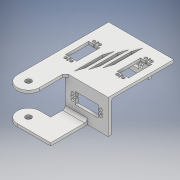
# Autodesk Inventor part: Rbiceps
Saved by Autodesk Inventor 2018 (Build 220112000, 112)
## iProperties
Created: 2018-02-07
Part Number: Rbiceps
Material: Plastique ABS
Document SubType Name: Modeling
Designer: Thomas
Density: 1.06 g/cm^3
Appearance: Lisse - Blanc
Mass: 118.74 g
Surface Area: 553.913 cm^2
Volume: 112.019 cm^3
Author: Thomas
Autodesk Inventor part; units mm, degrees
ref_plane "YZ Plane" through (0, 0, 0) normal (1, 0, 0) x (0, 1, 0)
ref_plane "XZ Plane" through (0, 0, 0) normal (0, 1, 0) x (-1, 0, 0)
ref_plane "XY Plane" through (0, 0, 0) normal (0, 0, 1) x (1, 0, 0)
sketch "Esquisse1" plane through (0, 0, 0) normal (0, 0, 1) x (1, 0, 0)
  line L0 (10, 0) -> (104.4, 0)
  line L1 (114.4, -10) -> (114.4, -105.15)
  line L2 (104.4, -115.15) -> (49, -115.15)
  line L3 (0, -115.15) -> (0, -10)
  line L4 (0, -115.15) -> (0, -160.65)
  line L5 (39, -160.65) -> (39, -125.15)
  arc A0 (0, -160.65) -> (39, -160.65) centre (19.5, -160.65) ccw
  line L6 (0, -10) -> (0, 0)
  line L7 (10, 0) -> (0, 0)
  line L8 (114.4, -10) -> (114.4, 0)
  line L9 (114.4, 0) -> (104.4, 0)
  line L10 (114.4, -105.15) -> (114.4, -115.15)
  line L11 (104.4, -115.15) -> (114.4, -115.15)
  line L12 (39, -125.15) -> (39, -115.15)
  line L13 (49, -115.15) -> (39, -115.15)
  dimension "d0" = 39
  dimension "d1" = 114.4
  dimension "d2" = 45.5
  dimension "d3" = 115.15
  constraints: 28 end point, 9 point on line, 5 vertical, 4 perpendicular, 2 horizontal, 2 parallel, 2 point on circle, 1 centre point
  measures "d0" distance of L4.end L5.start
  measures "d1" distance of L6.end L8.end
  measures "d2" distance of L5.start L12.end
  measures "d3" distance of L8.end L10.end
extrude "Extrusion1" add sketch "Esquisse1" along normal blind 5
sketch "Esquisse2" plane through (0, 0, 5) normal (0, 0, 1) x (1, 0, 0)
  line L0 (31.7, -46.85) -> (31.7, -87.85)
  line L1 (11.7, -87.85) -> (11.7, -46.85)
  line L2 (102.7, -26.7) -> (102.7, -67.7)
  line L3 (82.7, -67.7) -> (82.7, -26.7)
  line L4 (0, 0) -> (0, -160.65) projected
  line L5 (114.4, -115.15) -> (114.4, 0) projected
  circle A0 centre (16.7, -42.46) radius 2.5
  circle A1 centre (26.7, -42.46) radius 2.5
  circle A2 centre (16.7, -92.24) radius 2.5
  circle A3 centre (26.7, -92.24) radius 2.5
  circle A4 centre (87.7, -72.09) radius 2.5
  circle A5 centre (97.7, -72.09) radius 2.5
  circle A6 centre (87.7, -22.31) radius 2.5
  circle A7 centre (97.7, -22.31) radius 2.5
  circle A8 centre (19.5, -160.65) radius 5
  line L6 (114.4, 0) -> (0, 0) projected
  line L7 (39, -115.15) -> (114.4, -115.15) projected
  line L8 (22.7, -46.85) -> (22.7, -39.35)
  line L9 (22.7, -39.35) -> (20.7, -39.35)
  line L10 (20.7, -39.35) -> (20.7, -46.85)
  line L11 (93.7, -67.7) -> (93.7, -75.2)
  line L12 (91.7, -75.2) -> (91.7, -67.7)
  line L13 (93.7, -26.7) -> (93.7, -19.2)
  line L14 (93.7, -19.2) -> (91.7, -19.2)
  line L15 (91.7, -19.2) -> (91.7, -26.7)
  line L16 (11.7, -46.85) -> (20.7, -46.85)
  line L17 (31.7, -46.85) -> (22.7, -46.85)
  line L18 (22.7, -87.85) -> (22.7, -95.35)
  line L19 (22.7, -95.35) -> (20.7, -95.35)
  line L20 (20.7, -95.35) -> (20.7, -87.85)
  line L21 (11.7, -87.85) -> (20.7, -87.85)
  line L22 (22.7, -87.85) -> (31.7, -87.85)
  line L23 (82.7, -26.7) -> (91.7, -26.7)
  line L24 (93.7, -26.7) -> (102.7, -26.7)
  line L25 (82.7, -67.7) -> (91.7, -67.7)
  line L26 (93.7, -67.7) -> (102.7, -67.7)
  line L27 (91.7, -75.2) -> (93.7, -75.2)
  point P0 (0, -10)
  point P1 (114.4, -105.15)
  point P2 (114.4, -10)
  point P3 (39, -160.65)
  point P4 (104.4, 0)
  point P5 (10, 0)
  point P6 (49, -115.15)
  point P7 (104.4, -115.15)
  dimension "d7" = 11.7
  dimension "d8" = 11.7
  dimension "d9" = 20
  dimension "d10" = 20
  dimension "d11" = 41
  dimension "d12" = 41
  dimension "d13" = 10
  dimension "d14" = 19.5
  dimension "d16" = 5
  dimension "d18" = 5
  dimension "d20" = 10
  dimension "d21" = 5
  dimension "d22" = 5
  dimension "d26" = 10
  dimension "d28" = 5
  dimension "d31" = 5
  dimension "d32" = 10
  dimension "d33" = 5
  dimension "d36" = 5
  dimension "d37" = 10
  dimension "d41" = 9
  dimension "d43" = 4.39
  dimension "d44" = 4.39
  dimension "d45" = 5
  dimension "d46" = 7.5
  dimension "d47" = 7.5
  dimension "d48" = 9
  dimension "d49" = 9
  dimension "d50" = 9
  dimension "d51" = 5
  dimension "d52" = 4.39
  dimension "d53" = 4.39
  dimension "d54" = 7.5
  dimension "d55" = 9
  dimension "d56" = 9
  dimension "d57" = 4.39
  dimension "d58" = 4.39
  dimension "d59" = 5
  dimension "d60" = 9
  dimension "d61" = 9
  dimension "d62" = 7.5
  dimension "d63" = 4.39
  dimension "d64" = 4.39
  dimension "d65" = 5
  dimension "d168" = 41
  dimension "d169" = 41
  constraints: 48 end point, 9 centre point, 8 parallel, 4 horizontal, 3 collinear, 1 point on line
  measures "d7" distance between parallel lines of L1 L4
  measures "d8" distance between parallel lines of L5 L2
  measures "d9" distance of L0.end L1.start
  measures "d10" distance of L2.end L3.start
  measures "d11" distance of L0.start L0.end
  measures "d12" distance of L3.start L3.end
  measures "d13" diameter of A8
  measures "d14" distance of A8.centre point (39, -160.65)
  measures "d16" diameter of A2
  measures "d18" diameter of A3
  measures "d20" distance of A3.centre A2.centre
  measures "d21" diameter of A0
  measures "d22" diameter of A1
  measures "d26" distance of A1.centre A0.centre
  measures "d28" diameter of A5
  measures "d31" diameter of A4
  measures "d32" distance of A5.centre A4.centre
  measures "d33" diameter of A7
  measures "d36" diameter of A6
  measures "d37" distance of A7.centre A6.centre
  measures "d41" distance of L1.end L10.end
  measures "d43" distance from line of L16 A0.centre
  measures "d44" distance from line of L17 A1.centre
  measures "d45" horizontal distance of L1.end A0.centre
  measures "d46" distance of L8.start L8.end
  measures "d47" distance of L18.start L18.end
  measures "d48" distance of L1.start L20.end
  measures "d49" distance of L18.start L0.end
  measures "d50" distance of L0.start L8.start
  measures "d51" horizontal distance of A2.centre L1.start
  measures "d52" distance from line of L21 A2.centre
  measures "d53" distance from line of L22 A3.centre
  measures "d54" distance of L11.start L11.end
  measures "d55" distance of L3.start L12.end
  measures "d56" distance of L11.start L2.end
  measures "d57" distance from line of L25 A4.centre
  measures "d58" distance from line of L26 A5.centre
  measures "d59" distance from line of A4.centre L3
  measures "d60" distance of L3.end L15.end
  measures "d61" distance of L13.start L2.start
  measures "d62" distance of L14.end L15.end
  measures "d63" distance from line of L23 A6.centre
  measures "d64" distance from line of L24 A7.centre
  measures "d65" distance from line of L2 A7.centre
  measures "d168" distance of L1.start L1.end
  measures "d169" distance of L2.start L2.end
extrude "Extrusion2" cut sketch "Esquisse2" against normal blind 5
sketch "Esquisse3" plane through (39, -115.15, 0) normal (0, -1, 0) x (1, 0, 0)
  line L0 (0, 0) -> (75.4, 0) projected
  line L1 (0, 0) -> (75.4, 0)
  line L2 (75.4, 0) -> (75.4, -54.86)
  line L3 (75.4, -54.86) -> (0, -54.86)
  line L4 (0, -54.86) -> (0, 0)
  point P0 (-39, 0)
  dimension "d68" = 54.86
  constraints: 8 end point, 2 parallel, 1 horizontal, 1 perpendicular
  measures "d68" distance of L1.end L2.end
extrude "Extrusion3" add sketch "Esquisse3" against normal blind 5
sketch "Esquisse4" plane through (0, 0, 5) normal (0, 0, 1) x (1, 0, 0)
  line L0 (44.7, -55.15) -> (49.7, -40.15)
  line L1 (49.7, -40.15) -> (49.7, -90.15)
  line L2 (49.7, -90.15) -> (44.7, -105.15)
  line L3 (44.7, -105.15) -> (44.7, -55.15)
  line L4 (0, 0) -> (0, -160.65) projected
  line L5 (54.7, -40) -> (59.7, -25)
  line L6 (59.7, -25) -> (59.7, -75)
  line L7 (59.7, -75) -> (54.7, -90)
  line L8 (54.7, -90) -> (54.7, -40)
  line L9 (64.7, -25) -> (69.7, -10)
  line L10 (69.7, -10) -> (69.7, -60)
  line L11 (69.7, -60) -> (64.7, -75)
  line L12 (64.7, -75) -> (64.7, -25)
  line L13 (114.4, 0) -> (0, 0) projected
  line L14 (39, -115.15) -> (114.4, -115.15) projected
  dimension "d71" = 50
  dimension "d72" = 50
  dimension "d73" = 15
  dimension "d74" = 15
  dimension "d75" = 5
  dimension "d78" = 44.7
  dimension "d79" = 50
  dimension "d80" = 50
  dimension "d81" = 15
  dimension "d82" = 15
  dimension "d83" = 5
  dimension "d84" = 54.7
  dimension "d85" = 50
  dimension "d86" = 50
  dimension "d87" = 15
  dimension "d88" = 15
  dimension "d89" = 5
  dimension "d90" = 64.7
  dimension "d91" = 10
  dimension "d92" = 10
  dimension "d93" = 25
  constraints: 24 end point, 3 point on line, 3 vertical, 1 parallel
  measures "d71" distance of L0.end L1.end
  measures "d72" distance of L2.end L3.end
  measures "d73" vertical distance of L0.start L0.end
  measures "d74" vertical distance of L1.end L2.end
  measures "d75" distance from line of L1 L3.end
  measures "d78" distance between parallel lines of L4 L3
  measures "d79" distance of L5.end L6.end
  measures "d80" distance of L7.end L8.end
  measures "d81" vertical distance of L5.start L5.end
  measures "d82" vertical distance of L6.end L7.end
  measures "d83" distance from line of L6 L8.end
  measures "d84" distance between parallel lines of L4 L8
  measures "d85" distance of L9.end L10.end
  measures "d86" distance of L11.end L12.end
  measures "d87" vertical distance of L9.start L9.end
  measures "d88" vertical distance of L10.end L11.end
  measures "d89" distance from line of L10 L12.end
  measures "d90" distance between parallel lines of L4 L12
  measures "d91" distance from line of L13 L9.end
  measures "d92" distance from line of L14 L2.end
  measures "d93" distance from line of L13 L5.end
extrude "Extrusion4" cut sketch "Esquisse4" against normal blind 5
sketch "Esquisse5" plane through (39, -115.15, 5) normal (0, -1, 0) x (1, 0, 0)
  line L0 (17.2, -20) -> (58.2, -20)
  line L1 (58.2, -40) -> (17.2, -40)
  circle A0 centre (12.81, -25) radius 2.5
  circle A1 centre (12.81, -35) radius 2.5
  circle A2 centre (62.59, -25) radius 2.5
  circle A3 centre (62.59, -35) radius 2.5
  line L2 (0, 0) -> (75.4, 0) projected
  line L3 (0, -59.86) -> (0, -5) projected
  line L4 (17.2, -31) -> (9.7, -31)
  line L5 (9.7, -31) -> (9.7, -29)
  line L6 (9.7, -29) -> (17.2, -29)
  line L7 (58.2, -29) -> (65.7, -29)
  line L8 (65.7, -29) -> (65.7, -31)
  line L9 (65.7, -31) -> (58.2, -31)
  line L10 (17.2, -29) -> (17.2, -20)
  line L11 (17.2, -31) -> (17.2, -40)
  line L12 (58.2, -40) -> (58.2, -31)
  line L13 (58.2, -29) -> (58.2, -20)
  line L14 (75.4, -59.86) -> (75.4, 0) projected
  point P0 (-39, -5)
  dimension "d96" = 5
  dimension "d98" = 5
  dimension "d99" = 5
  dimension "d100" = 20
  dimension "d101" = 41
  dimension "d103" = 20
  dimension "d109" = 10
  dimension "d110" = 10
  dimension "d111" = 5
  dimension "d112" = 5
  dimension "d113" = 5
  dimension "d114" = 9
  dimension "d115" = 9
  dimension "d116" = 9
  dimension "d117" = 9
  dimension "d118" = 7.5
  dimension "d119" = 7.5
  dimension "d170" = 41
  dimension "d171" = 17.2
  dimension "d172" = 4.39
  dimension "d173" = 4.39
  dimension "d174" = 4.39
  dimension "d175" = 4.39
  dimension "d176" = 17.2
  constraints: 24 end point, 6 equal length, 4 centre point, 3 horizontal, 2 perpendicular, 1 vertical
  measures "d96" diameter of A1
  measures "d98" diameter of A2
  measures "d99" diameter of A3
  measures "d100" distance of L1.end L0.start
  measures "d101" distance of L0.start L0.end
  measures "d103" distance between parallel lines of L2 L0
  measures "d109" distance of A2.centre A3.centre
  measures "d110" distance of A0.centre A1.centre
  measures "d111" diameter of A0
  measures "d112" vertical distance of L0.start A0.centre
  measures "d113" vertical distance of A3.centre L1.start
  measures "d114" distance of L6.end L0.start
  measures "d115" distance of L4.start L1.end
  measures "d116" distance of L7.start L0.end
  measures "d117" distance of L1.start L9.end
  measures "d118" distance of L5.end L6.end
  measures "d119" distance of L7.start L7.end
  measures "d170" distance of L1.start L1.end
  measures "d171" distance between parallel lines of L3 L10
  measures "d172" distance from line of L13 A2.centre
  measures "d173" distance from line of L12 A3.centre
  measures "d174" distance from line of L11 A1.centre
  measures "d175" distance from line of L10 A0.centre
  measures "d176" distance between parallel lines of L14 L12
extrude "Extrusion5" cut sketch "Esquisse5" against normal blind 5
chamfer "Chanfrein1" distance 5 angle 45 1 edges at (39, -115.15, 2.5)
sketch "Esquisse7" plane through (114.4, -115.15, -54.86) normal (0, 0, -1) x (-1, 0, 0)
  line L0 (0, 0) -> (75.4, 0) projected
  line L1 (75.4, 0) -> (36.4, 0)
  line L2 (36.4, 0) -> (36.4, -65)
  line L3 (36.4, -65) -> (75.4, -65)
  line L4 (75.4, -65) -> (94.9, -65)
  arc A0 (94.9, -65) -> (94.9, -26) centre (94.9, -45.5) ccw
  line L5 (94.9, -26) -> (75.4, -26)
  line L6 (75.4, 0) -> (75.4, -26)
  point P0 (114.4, 115.15)
  dimension "d129" = 39
  dimension "d130" = 65
  dimension "d131" = 19.5
  constraints: 12 end point, 2 horizontal, 2 point on circle, 1 centre point, 1 coincident, 1 parallel, 1 perpendicular, 1 vertical
  measures "d129" distance of L2.end L3.end
  measures "d130" distance of L1.end L2.end
  measures "d131" distance of L3.end L4.end
extrude "Extrusion6" add sketch "Esquisse7" against normal blind 5
sketch "Esquisse8" plane through (114.4, -110.15, -54.86) normal (0, 0, -1) x (-1, 0, 0)
  circle A0 centre (94.9, -50.5) radius 5 projected
  circle A1 centre (94.9, -50.5) radius 5
  point P0 (114.4, 110.15)
  constraints: 1 centre point, 1 coincident
extrude "Extrusion7" cut sketch "Esquisse8" against normal blind 5
sketch "Esquisse9" plane through (0, 0, 0) normal (0, 1, 0) x (1, 0, 0)
  line L0 (0, 0) -> (75.4, 0)
  line L1 (75.4, 0) -> (75.4, 42.9)
  line L2 (75.4, 42.9) -> (0, 42.9)
  line L3 (0, 42.9) -> (0, 0)
  point P0 (114.4, 0)
  dimension "d137" = 39
  dimension "d138" = 42.9
  constraints: 8 end point, 2 parallel, 1 horizontal, 1 perpendicular
  measures "d137" distance of point (114.4, 0) L0.end
  measures "d138" distance of L2.end L0.start
extrude "Extrusion8" add sketch "Esquisse9" against normal blind 5
sketch "Esquisse10" plane through (0, 0, 5) normal (0, 1, 0) x (1, 0, 0)
  line L0 (58.2, 39.9) -> (17.2, 39.9)
  line L1 (17.2, 19.9) -> (58.2, 19.9)
  circle A0 centre (62.59, 34.9) radius 2.5
  circle A1 centre (62.59, 24.9) radius 2.5
  circle A2 centre (12.81, 34.9) radius 2.5
  circle A3 centre (12.81, 24.9) radius 2.5
  line L2 (75.4, 5) -> (75.4, 47.9) projected
  line L3 (58.2, 30.9) -> (65.7, 30.9)
  line L4 (65.7, 30.9) -> (65.7, 28.9)
  line L5 (65.7, 28.9) -> (58.2, 28.9)
  line L6 (17.2, 30.9) -> (9.7, 30.9)
  line L7 (9.7, 30.9) -> (9.7, 28.9)
  line L8 (9.7, 28.9) -> (17.2, 28.9)
  line L9 (58.2, 39.9) -> (58.2, 30.9)
  line L10 (58.2, 28.9) -> (58.2, 19.9)
  line L11 (17.2, 39.9) -> (17.2, 30.9)
  line L12 (17.2, 28.9) -> (17.2, 19.9)
  line L13 (0, 47.9) -> (0, 0) projected
  line L14 (75.4, 47.9) -> (0, 47.9) projected
  point P0 (0, 5)
  dimension "d141" = 41
  dimension "d142" = 20
  dimension "d143" = 5
  dimension "d144" = 5
  dimension "d145" = 5
  dimension "d146" = 5
  dimension "d151" = 10
  dimension "d152" = 5
  dimension "d154" = 10
  dimension "d156" = 5
  dimension "d157" = 9
  dimension "d158" = 9
  dimension "d159" = 7.5
  dimension "d160" = 7.5
  dimension "d161" = 17.2
  dimension "d162" = 17.2
  dimension "d163" = 4.39
  dimension "d164" = 17.2
  dimension "d167" = 8
  dimension "d177" = 4.39
  dimension "d178" = 4.39
  dimension "d179" = 4.39
  constraints: 24 end point, 5 equal length, 4 centre point, 3 horizontal, 3 perpendicular, 2 point on line, 1 vertical
  measures "d141" distance of L0.start L0.end
  measures "d142" distance of L0.end L1.start
  measures "d143" diameter of A0
  measures "d144" diameter of A1
  measures "d145" diameter of A2
  measures "d146" diameter of A3
  measures "d151" distance of A1.centre A0.centre
  measures "d152" vertical distance of A0.centre L0.start
  measures "d154" distance of A2.centre A3.centre
  measures "d156" distance from line of L0 A2.centre
  measures "d157" distance of L0.end L6.start
  measures "d158" distance of L8.end L1.start
  measures "d159" distance of L4.end L5.end
  measures "d160" distance of L7.end L8.end
  measures "d161" distance between parallel lines of L13 L11
  measures "d162" distance between parallel lines of L2 L10
  measures "d163" distance from line of L9 A0.centre
  measures "d164" distance between parallel lines of L13 L12
  measures "d167" distance between parallel lines of L0 L14
  measures "d177" distance from line of L11 A2.centre
  measures "d178" distance from line of L12 A3.centre
  measures "d179" distance from line of L10 A1.centre
extrude "Extrusion9" cut sketch "Esquisse10" against normal blind 5
fillet "Congé1" radius 5 1 edges at (37.7, -5, 0)
fillet "Congé2" radius 5 1 edges at (76.7, -110.15, 0)
fillet "Congé3" radius 5 1 edges at (58.5, -115.15, -49.86)
